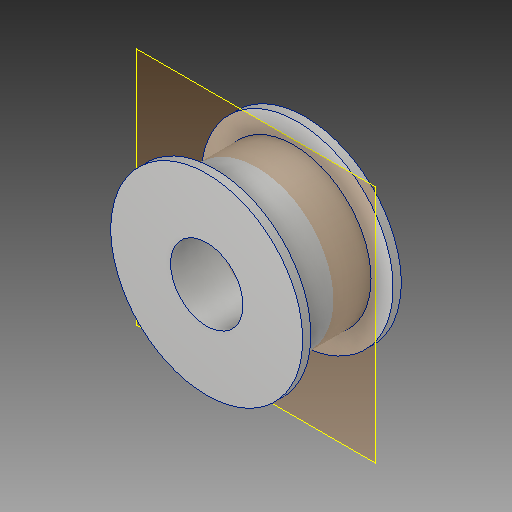
# Autodesk Inventor part: CAR_014_CarouselTensionerPulley
Saved by Autodesk Inventor 2018 (Build 220112000, 112)
## iProperties
Created: 2020-02-01
Part Number: CAR_014_CarouselTensionerPulley
Material: Aluminum 6061
Document SubType Name: Modeling
Designer: user
Mass: 46.6271 g
Surface Area: 66.6155 cm^2
Volume: 17.2693 cm^3
Density: 2.7 g/cm^3
Appearance: Aluminum - Flat
Author: user
Autodesk Inventor part; units mm, degrees
ref_plane "YZ Plane" through (0, 0, 0) normal (1, 0, 0) x (0, 1, 0)
ref_plane "XZ Plane" through (0, 0, 0) normal (0, 1, 0) x (-1, 0, 0)
ref_plane "XY Plane" through (0, 0, 0) normal (0, 0, 1) x (1, 0, 0)
sketch "Sketch1" plane through (0, 0, 0) normal (1, 0, 0) x (0, 1, 0)
  line L0 (0, 0) -> (16.9418, 0)
  line L1 (16.9418, 0) -> (16.9418, -16.4846)
  line L2 (16.9418, -16.4846) -> (0, -16.4846)
  line L3 (0, -16.4846) -> (0, 0)
  line L4 (21.0058, 2.54) -> (0, 2.54)
  line L5 (0, 2.54) -> (0, -19.0246)
  line L6 (0, -19.0246) -> (21.0058, -19.0246)
  line L7 (16.9418, 0) -> (21.0058, 0.762)
  line L8 (16.9418, -16.4846) -> (21.0058, -17.2466)
  line L9 (21.0058, -19.0246) -> (21.0058, -17.2466)
  line L10 (21.0058, 0.762) -> (21.0058, 2.54)
  dimension "d0" = 16.4846
  dimension "d2" = 2.54
  dimension "d3" = 2.54
  dimension "d5" = 1.778
  dimension "d6" = 1.778
  dimension "d7" = 4.064
  dimension "d8" = 4.064
  dimension "d10" = 21.0058
  constraints: 22 end point, 5 parallel, 2 horizontal, 2 perpendicular, 1 collinear
  measures "d0" distance of L0.end L1.end
  measures "d2" distance between parallel lines of L0 L4
  measures "d3" distance between parallel lines of L2 L6
  measures "d5" distance from line of L4 L7.end
  measures "d6" distance from line of L6 L8.end
  measures "d7" distance between parallel lines of L10 L1
  measures "d8" distance between parallel lines of L9 L1
  measures "d10" distance of L4.start L4.end
revolve "Revolution1" add sketch "Sketch1" angle 360 about axis through (0, 0, -16.4846) along (0, 0, 1)
sketch "Sketch2" plane through (0, 0, 2.54) normal (0, 0, 1) x (1, 0, 0)
  point P0 (0, 0)
  point P1 (0, 0)
  constraints: 1 coincident
hole "Hole1" at (0, 0, 2.54) direction (0, 0, -1) diameter 15.8496 end through all
ref_plane "Work Plane1" through (0, 0, -8.2423) normal (0, 0, 1) x (1, 0, 0)
equation "\"d8\" = d7"
body "Solid1"
